Autodesk Inventor part; units mm, degrees
(part 2 of 2)
  line L853 (-0.4714, 144.9681) -> (4.5286, 139.9681)
  line L854 (4.5286, 139.9681) -> (4.5286, -140.0318)
  line L855 (4.5286, -140.0318) -> (-0.4714, -145.0318)
  line L856 (-0.4714, -145.0318) -> (-30.4714, -145.0318)
  line L857 (-305.4714, -185.0318) -> (-310.4714, -180.2236)
  line L858 (-310.4714, -180.2236) -> (-310.4714, 179.9681)
  line L859 (-310.4714, 179.9681) -> (-305.4714, 184.9681)
  line L860 (-305.4714, 184.9681) -> (54.5286, 184.9681)
  line L861 (54.5286, 184.9681) -> (59.5286, 179.9681)
  line L862 (59.5286, 179.9681) -> (59.5286, -180.0318)
  line L863 (59.5286, -180.0318) -> (54.5286, -185.0318)
  line L864 (54.5286, -185.0318) -> (34.5286, -185.0318)
  line L865 (34.5286, -185.0318) -> (32.5286, -183.0318)
  line L866 (32.5286, -183.0318) -> (-283.4714, -183.0318)
  line L867 (-283.4714, -183.0318) -> (-285.4714, -185.0318)
  line L868 (-285.4714, -185.0318) -> (-305.4714, -185.0318)
  point P0 (0, 0)
  constraints: 1872 end point, 2 point on line
extrude "Extrusion1" add sketch "Sketch1" along normal blind 6
body "Solid1"
